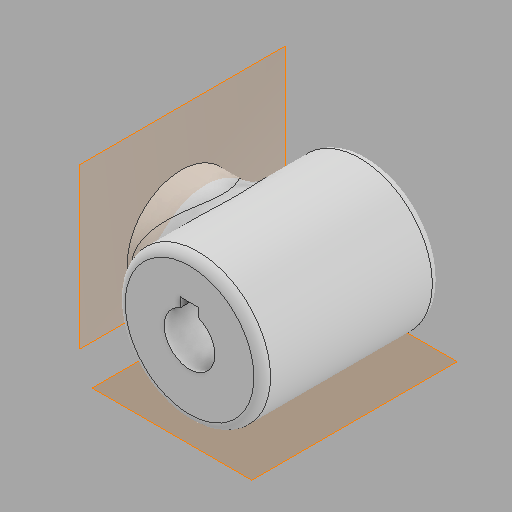
# Autodesk Inventor part: Крпеление ОУ
Saved by Autodesk Inventor 2025 (Build 290162000, 162)
## iProperties
Created: 2025-04-09
Part Number: Крпеление ОУ
Material: Типовые
Document SubType Name: Modeling
Designer: Artem Sannikov
Density: 1 g/cm^3
Appearance: По умолчанию
Author: Artem Sannikov
Autodesk Inventor part; units mm, degrees
ref_plane "РабПлоскость1" through (0, 0, 8.25) normal (0, 0, 1) x (1, 0, 0)
sketch "Эскиз1" plane through (0, 0, 8.25) normal (0, 0, 1) x (1, 0, 0)
  circle A0 centre (0, 0) radius 17.5
  circle A1 centre (0, 0) radius 6
  dimension "d1" = 35
  dimension "d2" = 12
  constraints: 2 centre point, 2 coincident
  measures "d1" diameter of A0
  measures "d2" diameter of A1
extrude "Выдавливание1" add sketch "Эскиз1" along normal blind 43
ref_plane "РабПлоскость2" through (0, -17.5, 8.25) normal (0, 1, 0) x (-1, 0, 0)
ref_plane "РабПлоскость3" through (-17.5, 0, 8.25) normal (1, 0, 0) x (0, 1, 0)
sketch "Эскиз2" plane through (-17.5, 0, 8.25) normal (1, 0, 0) x (0, 1, 0)
  line L0 (17.5, 43) -> (-17.5, 43) projected
  line L1 (0, 43) -> (0, 0) construction
  line L2 (17.5, 0) -> (-17.5, 0) projected
  circle A0 centre (0, 21.5) radius 13
  point P0 (0, -8.25)
  dimension "d23" = 26
  constraints: 3 midpoint, 2 end point, 1 centre point
  measures "d23" diameter of A0
extrude "Выдавливание2" add sketch "Эскиз2" along normal up to surface
sketch "Эскиз3" plane through (-17.5, 0, 8.25) normal (-1, 0, 0) x (0, 0, 1)
  arc A0 (8.5, 0) -> (34.5, 0) centre (21.5, 0) ccw construction
  circle A1 centre (21.5, 0) radius 13
  point P0 (-8.25, 0)
  point P1 (40, 0)
  point P2 (5, 0)
  point P3 (39, 0)
  point P4 (4, 0)
  point P5 (6.5, 0)
  point P6 (36.5, 0)
  constraints: 1 centre point, 1 coincident, 1 concentric
extrude "Выдавливание3" add sketch "Эскиз3" along normal blind 6
fillet "Сопряжение1" radius 5 3 edges at (-11.7154, -13, 29.7735) (-14.4476, 9.875, 21.2952) (-14.4454, 9.8782, 38.201)
fillet "Сопряжение2" radius 2 2 edges at (-17.5, 0, 8.25) (-17.5, 0, 51.25)
sketch "Эскиз5" plane through (-23.5, 0, 29.75) normal (-1, 0, 0) x (0, 0, 1)
  circle A0 centre (0, 0) radius 5
  circle A1 centre (0, 0) radius 10 construction
  circle A2 centre (0, 10) radius 2.2
  circle A3 centre (-7.8183, 6.2349) radius 2.2
  circle A4 centre (-9.7493, -2.2252) radius 2.2
  circle A5 centre (-4.3388, -9.0097) radius 2.2
  circle A6 centre (4.3388, -9.0097) radius 2.2
  circle A7 centre (9.7493, -2.2252) radius 2.2
  circle A8 centre (7.8183, 6.2349) radius 2.2
  point P0 (-29.75, 0)
  dimension "d17" = 20
  dimension "d14" = 10
  dimension "d18" = 4.4
  dimension "d21" = 360
  constraints: 8 centre point, 1 coincident, 1 vertical alignment, 17 other
  measures "d14" diameter of A0
  measures "d18" diameter of A2
extrude "Выдавливание5" cut sketch "Эскиз5" against normal blind 15.5
sketch "Эскиз6" plane through (0, 0, 8.25) normal (0, 0, -1) x (-1, 0, 0)
  line L0 (-2.1, 2.2009) -> (2.1, 2.2009)
  line L1 (2.1, 2.2009) -> (2.1, 7.8)
  line L2 (2.1, 7.8) -> (-2.1, 7.8)
  line L3 (-2.1, 7.8) -> (-2.1, 2.2009)
  line L4 (-2.1, 2.2009) -> (2.1, 7.8) construction
  line L5 (2.1, 2.2009) -> (-2.1, 7.8) construction
  circle A0 centre (0, 0) radius 6 projected
  point P0 (0, 5.0005)
  point P1 (-2.1, 5.6205)
  point P2 (2.1, 5.6205)
  dimension "d24" = 4.2
  dimension "d25" = 7.8
  constraints: 12 end point, 2 midpoint, 2 parallel, 1 horizontal, 1 perpendicular
  measures "d24" distance of L1.end L2.end
  measures "d25" distance from line of L2 A0.centre
extrude "Выдавливание6" cut sketch "Эскиз6" against normal through all contours L3 L2 L1 A0
sketch "Эскиз7" plane through (0, 0, 51.25) normal (0, 0, 1) x (1, 0, 0)
  arc A0 (-2.1, 5.6205) -> (2.1, 5.6205) centre (0, 0) ccw construction
  line L0 (2.1, 7.8) -> (2.1, 5.6205) construction
  line L1 (-2.1, 5.6205) -> (-2.1, 7.8) construction
  line L2 (-2.1, 7.8) -> (2.1, 7.8) construction
  arc A1 (-2.2, 5.6895) -> (2.2, 5.6895) centre (0, 0) ccw
  line L3 (-2.2, 5.6895) -> (-2.2, 7.9)
  line L4 (-2.2, 7.9) -> (2.2, 7.9)
  line L5 (2.2, 7.9) -> (2.2, 5.6895)
  dimension "d28" = 0.1
  constraints: 6 end point, 2 point on circle, 1 centre point, 3 other
  measures "d28" radial gap between concentric circles of A0 A1
extrude "Выдавливание7" cut sketch "Эскиз7" against normal blind 56.75
